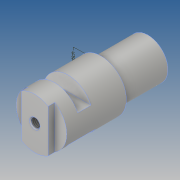
# Autodesk Inventor part: 200-20-ROCKER-CONNECTOR-01
Saved by Autodesk Inventor 2018.2 (Build 222227000, 227)
## iProperties
Manager: feesmrt
Company: FRANC0R
Created: 2017-10-30
Part Number: 200-20-ROCKER-CONNECTOR-01
Material: Aluminium 6061
Document SubType Name: Modeling
Designer: feesmrt
Density: 2.7 g/cm^3
Appearance: Aluminium - flach
Project: Rescue Robot
Cost Center: -
Description: Rocker Profile Connector
Engineer: feesmrt
Authority: feesmrt
Stock Number: 200-20-ROCKER-CONNECTOR-01
Mass: 197.92 g
Surface Area: 134.643 cm^2
Volume: 73.3037 cm^3
Author: feesmrt
Title: Rocker Profile Connector
Subject: Rescue Robot
Revision Number: 1
Autodesk Inventor part; units mm, degrees
ref_plane "YZ Plane" through (0, 0, 0) normal (1, 0, 0) x (0, 1, 0)
ref_plane "XZ Plane" through (0, 0, 0) normal (0, 1, 0) x (-1, 0, 0)
ref_plane "XY Plane" through (0, 0, 0) normal (0, 0, 1) x (1, 0, 0)
derived "200-10-ROCKER-BEARING-01.ipt"
sketch "Skizze_Lagersitz" plane through (0, 0, 0) normal (1, 0, 0) x (0, 1, 0)
  line L0 (-12.5, 36) -> (17.5, 36)
  line L1 (-12.5, -36) -> (-12.5, 36)
  line L2 (-17.5, 32.25) -> (-12.5, 32.25)
  line L3 (-17.5, -32.25) -> (-17.5, 32.25)
  line L4 (-32.5, 18) -> (-17.5, 18)
  line L5 (-32.5, -18) -> (-17.5, -18)
  line L6 (-17.5, -32.25) -> (-12.5, -32.25)
  line L7 (-12.5, -36) -> (17.5, -36)
  line L8 (32.5, 50) -> (32.5, -50)
  line L9 (30, -50) -> (30, 0)
  line L10 (-32.5, -18) -> (-32.5, 18)
  line L11 (-32.5, 50) -> (-32.5, -50)
  line L12 (-32.5, -50) -> (-32.5, 50)
  line L13 (-12.5, -36) -> (-12.5, 36)
  line L14 (17.5, -37.5) -> (17.5, 37.5)
  line L15 (17.5, 37.5) -> (32.5, 37.5)
  point P0 (0, 0)
  point P1 (30, 86)
  point P2 (30, 14)
  point P3 (-30, 32)
  point P4 (-30, 68)
  point P5 (32.5, 36)
  point P6 (32.5, -36)
sketch "Skizze4" plane through (0, 0, 0) normal (1, 0, 0) x (0, 1, 0)
  line L0 (-81.26, 0) -> (51.46, 0) projected
  line L1 (-12.5, -36) -> (-12.5, 36) construction
  line L2 (-32.5, -18) -> (-32.5, 18) construction
  line L3 (22.7, 0) -> (22.7, 15)
  line L4 (22.7, 15) -> (-12.5, 15)
  line L5 (17.7, 0) -> (17.7, 36) construction
  line L6 (-12.5, 15) -> (-12.5, 19)
  line L7 (-12.5, 19) -> (-62.3, 19)
  line L8 (-62.3, 0) -> (22.7, 0)
  line L9 (-62.3, 19) -> (-62.3, 0)
  line L10 (-12.5, 36) -> (17.5, 36) construction
  point P0 (0, 0)
  dimension "d3" = 30.2
  dimension "d4" = 5
  dimension "d5" = 30
  dimension "d6" = 38
  dimension "d7" = 85
  constraints: 14 end point, 6 point on line, 2 horizontal, 2 vertical, 1 collinear, 1 perpendicular
  measures "d3" distance between parallel lines of L5 L1
  measures "d4" distance between parallel lines of L3 L5
  measures "d5" diameter of L4 L0
  measures "d6" diameter of L7 L0
  measures "d7" distance from line of L7.end L3
revolve "Grundkoerper" add sketch "Skizze4" angle 360 about axis through (0, 0, 0) along (0, 1, 0)
sketch "Skizze11" plane through (0, -62.3, 0) normal (0, -1, 0) x (1, 0, 0)
  circle A0 centre (0, 0) radius 19 projected
hole "M6x12_CubeConn" at (0, -62.3, 0) direction (0, 1, 0) diameter 6.647 depth 25 tip angle 118 countersink diameter 8 countersink angle 90 thread size "M8x1.25" class "6H" standard "ISO Metric profile"
sketch "Skizze14" plane through (0, 22.7, 0) normal (0, 1, 0) x (1, 0, 0)
  circle A0 centre (0, 0) radius 15 construction
  constraints: 1 coincident
hole "M6x12_BearingFix" at (0, 22.7, 0) direction (0, -1, 0) diameter 4.917 depth 17.1 tip angle 118 countersink diameter 6 countersink angle 90 thread size "M6x1" class "6H" standard "ISO Metric profile"
sketch "Skizze15" plane through (0, 0, 0) normal (1, 0, 0) x (0, 1, 0)
  line L0 (-62.3, 19) -> (-12.5, 19) construction
  line L1 (-81.26, 0) -> (51.46, 0) projected
  line L2 (-62.3, -19) -> (-62.3, 19) construction
  line L3 (-12.5, -19) -> (-12.5, 19) construction
  line L4 (-47.3, 19) -> (-47.3, 8)
  line L5 (-47.3, 8) -> (-37.3, 8)
  line L6 (-37.3, 8) -> (-37.3, 19)
  line L7 (-42.3, 19) -> (-42.3, -19) construction
  line L8 (-62.3, -19) -> (-12.5, -19) projected
  line L9 (-47.3, 19) -> (-37.3, 19)
  line L10 (-62.3, -19) -> (-12.5, -19) projected
  line L11 (-52.3, -19) -> (-52.3, -11)
  line L12 (-62.3, -19) -> (-12.5, -19) projected
  line L13 (-52.3, -11) -> (-32.3, -11)
  line L14 (-32.3, -11) -> (-32.3, -19)
  line L15 (-62.3, -19) -> (-12.5, -19) projected
  line L16 (-32.3, -19) -> (-52.3, -19)
  line L17 (-62.3, -19) -> (-12.5, -19) projected
  point P0 (0, 0)
  dimension "d103" = 20
  dimension "d104" = 10
  dimension "d105" = 11
  dimension "d115" = 8
  dimension "d116" = 20
  constraints: 18 end point, 6 perpendicular, 5 point on line, 2 vertical, 1 horizontal, 5 other
  measures "d103" distance between parallel lines of L2 L7
  measures "d104" distance of L4.end L5.end
  measures "d105" distance between parallel lines of L0 L5
  measures "d115" distance between parallel lines of L16 L13
  measures "d116" distance of L11.end L13.end
extrude "Absatz_M8" cut sketch "Skizze15" along normal through all both and the other way through all
sketch "Skizze16" plane through (-17.2337, -47.3, 8) normal (0, 0, 1) x (1, 0, 0)
  line L0 (17.2337, 98.76) -> (17.2337, -33.96) construction
  line L1 (0, 0) -> (34.4674, 0) construction
  line L2 (34.4674, 10) -> (0, 10) construction
  line L3 (0, 0) -> (34.4674, 0) projected
  line L4 (17.2337, 0) -> (17.2337, 10) construction
  point P0 (17.2337, 47.3)
  point P1 (17.2337, 5)
  constraints: 3 midpoint, 2 end point
hole "D6_Boh" at (0, -42.3, 8) direction (0, 0, -1) diameter 6 end through all
sketch "Skizze17" plane through (0, -62.3, 0) normal (0, -1, 0) x (1, 0, 0)
  circle A0 centre (0, 0) radius 19 projected
  line L0 (-26.6, 0) -> (26.6, 0) construction
  line L1 (0, 113.2) -> (0, -77.2) construction
  arc A1 (17.2337, 8) -> (-17.2337, 8) centre (0, 0) ccw projected
  arc A2 (-15.4919, -11) -> (15.4919, -11) centre (0, 0) ccw projected
  line L2 (-10, 16.1555) -> (-10, -16.1555)
  line L3 (10, 16.1555) -> (10, -16.1555)
  dimension "d120" = 20
  constraints: 4 end point, 2 vertical, 6 other
  measures "d120" distance between parallel lines of L2 L3
extrude "Absatz_Torsionssicherung" cut sketch "Skizze17" against normal blind 5 contours A0 L3 | L2 A0
